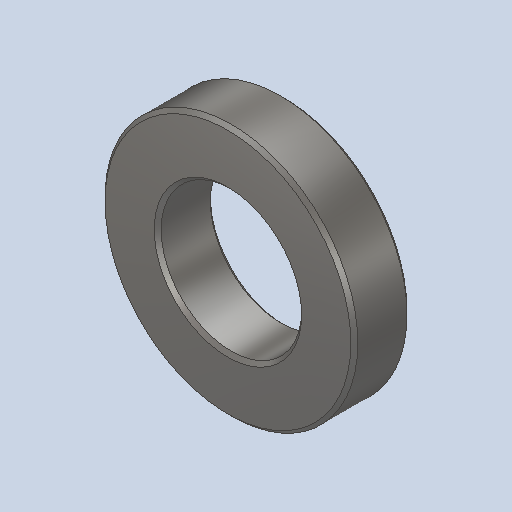
# Autodesk Inventor part: 1_250_ID_x_2_250_OD_X_0_500_Radial_Bearing_EE11S-2RS
Saved by Autodesk Inventor 2022.3 (Build 263350000, 350)
## iProperties
Created: 2023-01-21
Part Number: 1_250_ID_x_2_250_OD_X_0_500_Radial_Bearing_EE11S-2RS
Material: Steel, Mild
Document SubType Name: Modeling
Designer: mavericks
Density: 7.85 g/cm^3
Appearance: Semi-Polished
Mass: 175.43 g
Surface Area: 68.346 cm^2
Volume: 22.3477 cm^3
Author: mavericks
Autodesk Inventor part; units mm, degrees
ref_plane "YZ Plane" through (0, 0, 0) normal (1, 0, 0) x (0, 1, 0)
ref_plane "XZ Plane" through (0, 0, 0) normal (0, 1, 0) x (-1, 0, 0)
ref_plane "XY Plane" through (0, 0, 0) normal (0, 0, 1) x (1, 0, 0)
sketch "Sketch1" plane through (0, 0, 0) normal (0, 0, 1) x (1, 0, 0)
  circle A0 centre (0, 0) radius 28.575
  circle A1 centre (0, 0) radius 15.875
  dimension "d0" = 57.15
  dimension "d1" = 31.75
  constraints: 2 centre point, 2 coincident
  measures "d0" diameter of A0
  measures "d1" diameter of A1
extrude "Extrusion1" add sketch "Sketch1" along normal blind 12.7
chamfer "Chamfer1" distance 0.7925 angle 45 4 edges at (-15.875, 0, 12.7) (-15.875, 0, 0) (-28.575, 0, 12.7) (-28.575, 0, 0)
body "Solid1"
